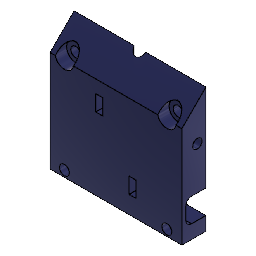
1-tensioner_mount_bracket v2 (Autodesk Fusion 360 design; units mm, degrees)
Autodesk Fusion 360 part; units mm, degrees
note: some values were not read from the file. Set by a fixed rule: which face or edge a step refers to.
sketch "Main Profile" plane through (0, 0, 0) normal (0, 1, 0) x (1, 0, 0)
  line L0 (-23.25, -44.1) -> (23.25, -44.1)
  line L1 (23.25, -44.1) -> (23.25, 0)
  line L2 (23.25, 0) -> (-23.25, 0)
  line L3 (-23.25, 0) -> (-23.25, -44.1)
  circle A0 centre (-18.15, -36.25) radius 3.25
  circle A1 centre (-18.15, -36.25) radius 1.75
  circle A2 centre (17.95, -36.25) radius 1.75
  circle A3 centre (17.95, -36.25) radius 3.25
  circle A4 centre (-18.15, -2.25) radius 1.75
  circle A5 centre (17.95, -2.25) radius 1.75
  line L4 (-7.09, -25.525) -> (-4.64, -25.525)
  line L5 (-4.64, -25.525) -> (-4.64, -31.1)
  line L6 (-4.64, -31.1) -> (-7.09, -31.1)
  line L7 (-7.09, -31.1) -> (-7.09, -25.525)
  line L8 (7.09, -11.805) -> (4.64, -11.805)
  line L9 (7.09, -6.23) -> (7.09, -11.805)
  line L10 (4.64, -11.805) -> (4.64, -6.23)
  line L11 (4.64, -6.23) -> (7.09, -6.23)
  point P0 (0, -18.665)
  dimension "d1" = 46.5
  dimension "d2" = 44.1
  dimension "d5" = 6.5
  dimension "d6" = 3.5
  dimension "d7" = 5.1
  dimension "d8" = 7.85
  dimension "d11" = 36.1
  dimension "d12" = 0
  dimension "d15" = 0
  dimension "d16" = 34
  dimension "d17" = 5.575
  dimension "d18" = 2.45
  dimension "d19" = 13
  dimension "d20" = 16.16
  dimension "d22" = 360
  dimension "d23" = 18.665
  constraint horizontal L0
  constraint vertical L1
  constraint horizontal L2
  constraint vertical L3
  constraint midpoint origin L2
  constraint concentric A0 A1
  constraint horizontal L4
  constraint vertical L5
  constraint horizontal L6
  constraint vertical L7
  constraint vertical origin P0
  measures "d1" distance of L0.start L0.end
  measures "d2" distance of L0.start L2.end
  measures "d5" diameter of A0
  measures "d6" diameter of A1
  measures "d7" distance of L3 A0.centre
  measures "d8" distance of L0 A0.centre
  measures "d17" distance of L4 L6
  measures "d18" distance of L5 L7
  measures "d19" distance of L0 L6
  measures "d20" distance of L3 L7
  measures "d23" distance of origin P0
extrude "Extrude1" add sketch "Main Profile" against normal blind 8.5 contours L0 L1 L2 L3 makes body 1
extrude "Extrude2" add sketch "Main Profile" against normal blind 4.5 contours A0 | A3 bodies 1
chamfer "Chamfer1" distance 8.5 angle 45 1 edges at (0, -8.5, 44.1) on bodies 1
sketch "Side" plane through (23.25, 0, 0) normal (1, 0, 0) x (0, 1, 0)
  line L0 (0, 44.1) -> (-8.5, 35.6)
  line L1 (-8.5, 35.6) -> (-8.5, 0)
  line L2 (-8.5, 0) -> (0, 0)
  line L3 (0, 0) -> (0, 44.1)
  line L4 (0, 13.22) -> (-7.12, 13.22)
  line L5 (-7.12, 13.22) -> (-7.12, 4.87)
  line L6 (-7.12, 4.87) -> (0, 4.87)
  line L7 (0, 4.87) -> (0, 13.22)
  circle A0 centre (-3.05, 9.045) radius 1.65
  line L8 (-7.12, 9.045) -> (0, 9.045) construction
  dimension "d29" = 8.35
  dimension "d30" = 7.12
  dimension "d31" = 4.87
  dimension "d32" = 3.3
  dimension "d33" = 3.05
  constraint horizontal L4
  constraint vertical L5
  constraint horizontal L6
  constraint vertical L7
  constraint coincident L3 L4.start
  constraint midpoint L5 L8.start
  constraint midpoint L7 L8.end
  constraint coincident A0.centre L8
  measures "d29" distance of L4 L6
  measures "d30" distance of L4.start L4.end
  measures "d31" distance of L2 L6
  measures "d32" diameter of A0
  measures "d33" distance of L7 A0.centre
extrude "Extrude3" add sketch "Side" against normal blind 43.75 separate body contours A0 makes body 2
extrude "Extrude4" add sketch "Side" against normal blind 12 contours L3 L4 L5 L6 L7 bodies 2
copy_body "CopyPasteBodies1" bodies 2 makes body 3
move_body "Move1" bodies 3 to x (-1, 0, 0) y (0, 1, 0) z (0, 0, -1) at (0, 0, 37.35)
combine "Combine1" operation cut target body 1 tool bodies 2 3
fillet "Fillet1" radius 2 4 edges at (17.25, -7.12, 13.22) (-17.25, -7.12, 32.48) (-17.25, -7.12, 24.13) (17.25, -7.12, 4.87) on bodies 1
sketch "Sketch3" plane through (0, 0, 0) normal (0, 0, -1) x (1, 0, 0)
  line L0 (-23.25, 0) -> (23.25, 0)
  line L1 (23.25, 0) -> (23.25, 8.5)
  line L2 (23.25, 8.5) -> (-23.25, 8.5)
  line L3 (-23.25, 8.5) -> (-23.25, 0)
  arc A0 (2.0331, 0) -> (-2.0331, 0) centre (0, -0.5259) ccw
  dimension "d40" = 2.1
  constraint coincident L0 A0.start
  constraint coincident L0 A0.end
  constraint vertical origin A0.centre
  measures "d40" radius of A0
extrude "Extrude5" cut sketch "Sketch3" against normal blind 53.766 contours L0 A0 bodies 1
extrude "Extrude6" cut 1 faces at (20.5, -2.5061, 28.387) along direction (1, 0, 0) blind 10 on bodies 1 bodies 1
extrude "Extrude7" cut 1 faces at (-20.5, -2.4761, 8.8865) along direction (-1, 0, 0) blind 20 on bodies 1 bodies 1
named bodies: "1-tensioner_mount_bracket", "Tool", "Tool (1)"
